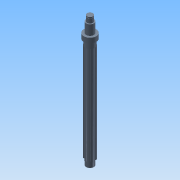
# Autodesk Inventor part: 主动轴
Saved by Autodesk Inventor 2015 (Build 190159000, 159)
## iProperties
Created: 2017-05-09
Part Number: 主动轴
Material: 常规
Document SubType Name: Modeling
Designer: Administrator
Density: 1 g/cm^3
Appearance: 钢蓝色
Author: Administrator
Autodesk Inventor part; units mm, degrees
ref_plane "YZ Plane" through (0, 0, 0) normal (1, 0, 0) x (0, 1, 0)
ref_plane "XY Plane" through (0, 0, 0) normal (0, 0, 1) x (1, 0, 0)
sketch "草图1" plane through (0, 0, 0) normal (0, 0, 1) x (1, 0, 0)
  circle A0 centre (0, 0) radius 32
  dimension "d0" = 64
  constraints: 1 centre point, 1 coincident
  measures "d0" diameter of A0
extrude "拉伸1" add sketch "草图1" along normal blind 25
sketch "草图2" plane through (0, 0, 25) normal (0, 0, 1) x (1, 0, 0)
  circle A0 centre (0, 0) radius 20
  dimension "d3" = 40
  constraints: 1 centre point, 1 coincident
  measures "d3" diameter of A0
extrude "拉伸2" add sketch "草图2" along normal blind 80
sketch "草图3" plane through (0, 0, 0) normal (0, 0, -1) x (-1, 0, 0)
  circle A0 centre (0, 0) radius 25
  dimension "d6" = 50
  constraints: 1 centre point, 1 coincident
  measures "d6" diameter of A0
extrude "拉伸3" add sketch "草图3" along normal blind 535
sketch "草图4" plane through (0, 0, -535) normal (0, 0, -1) x (-1, 0, 0)
  circle A0 centre (0, 0) radius 20
  dimension "d9" = 40
  constraints: 1 centre point, 1 coincident
  measures "d9" diameter of A0
extrude "拉伸4" add sketch "草图4" along normal blind 30
chamfer "倒角1" distance 2 angle 45 1 edges at (20, 0, -565)
sketch "草图5" plane through (0, 0, -535) normal (0, 0, -1) x (-1, 0, 0)
  circle A0 centre (0, 0) radius 25
  circle A1 centre (0, 0) radius 20
  line L0 (-4, 24.6779) -> (-4, 19.5959)
  line L1 (4, 24.6779) -> (4, 19.5959)
  circle A2 centre (0, 0) radius 20 projected
  circle A3 centre (0, 0) radius 25 projected
  line L2 (0, 0) -> (0, 7.2531)
  line L3 (-19.3717, 15.8031) -> (-14.9706, 13.2621)
  line L4 (-23.3717, -8.8749) -> (-18.9706, -6.3339)
  line L5 (-4, -24.6779) -> (-4, -19.5959)
  line L6 (19.3717, -15.8031) -> (14.9706, -13.2621)
  line L7 (23.3717, 8.8749) -> (18.9706, 6.3339)
  line L8 (-14.9706, 13.2621) -> (-19.3717, 15.8031)
  arc A4 (-4, 24.6779) -> (-19.3717, 15.8031) centre (0, 0) ccw
  arc A5 (-4, 19.5959) -> (-14.9706, 13.2621) centre (0, 0) ccw
  dimension "d15" = 50
  dimension "d16" = 40
  dimension "d17" = 7.2531
  dimension "d18" = 4
  dimension "d19" = 8
  dimension "d22" = 360
  constraints: 18 end point, 6 point on circle, 3 centre point, 3 vertical, 2 coincident, 2 parallel, 1 collinear, 24 other
  measures "d16" diameter of A1
  measures "d17" distance of L2.start L2.end
  measures "d18" distance between parallel lines of L2 L0
  measures "d19" distance between parallel lines of L1 L0
extrude "拉伸5" cut sketch "草图5" against normal blind 505 contours L0 A1 L3 A0
pattern_circular "环形阵列1" count 6 over 360 about axis through (0, 0, -10) along (0, 0, 1) of "拉伸5"
sketch "草图6" plane through (0, 0, 105) normal (0, 0, 1) x (1, 0, 0)
  circle A0 centre (0, 0) radius 15
  circle A1 centre (0, 0) radius 20
  dimension "d29" = 30
  dimension "d30" = 40
  constraints: 2 centre point, 2 coincident
  measures "d29" diameter of A0
  measures "d30" diameter of A1
extrude "拉伸6" cut sketch "草图6" against normal blind 28.578
sketch "草图7" plane through (0, 0, 0) normal (0, 1, 0) x (-1, 0, 0)
  line L0 (-13.95, 99.352) -> (-18.95, 99.352)
  line L1 (-18.95, 99.352) -> (-18.95, 100.752)
  line L2 (-18.95, 100.752) -> (-13.95, 100.752)
  line L3 (-13.95, 100.752) -> (-13.95, 99.352)
  line L4 (0, 0) -> (0, 169.8002)
  line L5 (15, 105) -> (-15, 105) projected
  line L6 (0, -711.96) -> (0, 316.7602) projected
  dimension "d33" = 169.8002
  dimension "d34" = 13.95
  dimension "d35" = 4.248
  dimension "d36" = 1.4
  dimension "d37" = 5
  constraints: 10 end point, 2 parallel, 1 horizontal, 1 perpendicular, 1 vertical
  measures "d33" distance of L4.start L4.end
  measures "d34" distance between parallel lines of L4 L3
  measures "d35" distance between parallel lines of L5 L2
  measures "d36" distance of L0.end L1.end
  measures "d37" distance of L0.start L0.end
revolve "旋转1" cut sketch "草图7" angle 360 about axis through (0, 0, -10) along (0, 0, 1)
ref_plane "工作平面1" through (0, 15, 105) normal (0, 1, 0) x (-1, 0, 0)
sketch "草图8" plane through (0, 15, 105) normal (0, 1, 0) x (-1, 0, 0)
  line L0 (4, -22.237) -> (-4, -22.237)
  line L1 (-4, -22.237) -> (-4, -12.237)
  line L2 (-4, -12.237) -> (4, -12.237)
  line L3 (4, -12.237) -> (4, -22.237)
  arc A0 (-4, -22.237) -> (4, -22.237) centre (0, -22.237) ccw
  arc A1 (4, -12.237) -> (-4, -12.237) centre (0, -12.237) ccw
  line L4 (-15, -5.648) -> (15, -5.648) projected
  line L5 (15, 0) -> (-15, 0) projected
  line L6 (0, 0) -> (0, 18.2304)
  point P0 (0, -105)
  dimension "d39" = 8
  dimension "d40" = 10
  dimension "d41" = 6.589
  dimension "d42" = 18.2304
  constraints: 10 end point, 4 point on circle, 4 tangent, 2 centre point, 2 midpoint, 2 parallel, 1 horizontal, 1 perpendicular, 1 point on line, 1 vertical
  measures "d39" distance of L0.start L0.end
  measures "d40" distance of L0.end L1.end
  measures "d41" distance between parallel lines of L2 L4
  measures "d42" distance of L6.start L6.end
extrude "拉伸7" cut sketch "草图8" against normal blind 3
